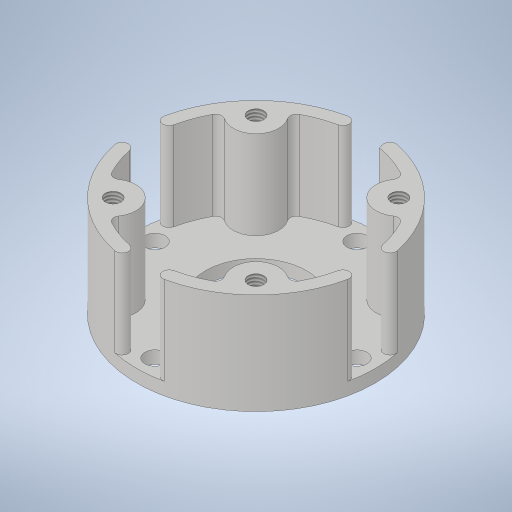
# Autodesk Inventor part: NEO MOUNT
Saved by Autodesk Inventor 2023.3 (Build 273359000, 359)
## iProperties
Created: 2024-01-28
Part Number: NEO MOUNT
Material: Generic
Document SubType Name: Modeling
Designer: mavericks
Density: 1 g/cm^3
Appearance: Default
Author: mavericks
Autodesk Inventor part; units mm, degrees
ref_plane "YZ Plane" through (0, 0, 0) normal (1, 0, 0) x (0, 1, 0)
ref_plane "XZ Plane" through (0, 0, 0) normal (0, 1, 0) x (-1, 0, 0)
ref_plane "XY Plane" through (0, 0, 0) normal (0, 0, 1) x (1, 0, 0)
sketch "Sketch1" plane through (0, 0, 0) normal (0, 1, 0) x (-1, 0, 0)
  circle A0 centre (0, 0) radius 25.4
  circle A1 centre (0, 0) radius 29.972
  dimension "d0" = 50.8
  dimension "d1" = 59.944
  constraints: 2 centre point, 2 coincident
  measures "d0" diameter of A0
  measures "d1" diameter of A1
extrude "Extrusion1" add sketch "Sketch1" along normal blind 3.175 contours A0 | A1
sketch "Sketch2" plane through (0, 3.175, 0) normal (0, 1, 0) x (1, 0, 0)
  circle A0 centre (0, 0) radius 25.4
  point P0 (-25.4, 0)
  point P1 (-17.9605, -17.9605)
  point P2 (0, -25.4)
  point P3 (17.9605, -17.9605)
  point P4 (25.4, 0)
  point P5 (17.9605, 17.9605)
  point P6 (0, 25.4)
  point P7 (-17.9605, 17.9605)
  dimension "d4" = 50.8
  dimension "d7" = 360
  constraints: 2 horizontal alignment, 1 coincident, 11 other
hole "Hole1" at (-25.4, 3.175, 0) at (0, 3.175, 25.4) at (25.4, 3.175, 0) at (0, 3.175, -25.4) direction (0, -1, 0) diameter 5.1054 end through all clearance for "Flat Head Machine Screw (82)" size "#10" standard "Ansi Unified Screw Threads"
sketch "Sketch3" plane through (0, 3.175, 0) normal (0, 1, 0) x (1, 0, 0)
  circle A0 centre (0, 0) radius 29.972 projected
  circle A1 centre (0, 0) radius 26.797
  circle A2 centre (-17.9605, -17.9605) radius 5.7277
  circle A3 centre (-17.9605, 17.9605) radius 5.7277
  circle A4 centre (17.9605, 17.9605) radius 5.7277
  circle A5 centre (17.9605, -17.9605) radius 5.7277
  circle A6 centre (25.4, 0) radius 2.5527 projected
  circle A7 centre (-25.4, 0) radius 2.5527 projected
  circle A8 centre (0, -25.4) radius 2.5527 projected
  circle A9 centre (0, 25.4) radius 2.5527 projected
  circle A10 centre (0, 0) radius 29.972 projected
  point P0 (-22.5303, -14.5074)
  point P1 (-22.5303, 14.5074)
  point P2 (-14.5074, 22.5303)
  point P3 (14.5074, 22.5303)
  point P4 (22.5303, 14.5074)
  point P5 (22.5303, -14.5074)
  point P6 (14.5074, -22.5303)
  point P7 (-14.5074, -22.5303)
  point P8 (-26.7071, -2.1926)
  point P9 (-26.7071, 2.1926)
  point P10 (-2.1926, 26.7071)
  point P11 (2.1926, 26.7071)
  point P12 (26.7071, 2.1926)
  point P13 (26.7071, -2.1926)
  point P14 (2.1926, -26.7071)
  point P15 (-2.1926, -26.7071)
  dimension "d16" = 3.175
  constraints: 5 centre point
  measures "d16" radial gap between concentric circles of A0 A1
extrude "Extrusion2" add sketch "Sketch3" along normal blind 22.225 contours A0 A5 A1 A6 A4 | A4 A1 A0 | A0 A5 A1 | A4 A1 A9 A3 A0 | A0 A2 A1 A8 A5 | A3 A1 A0 | A1 A4 | A0 A2 A1 | A5 A1 | A3 A1 A7 A2 A0 | A3 A1 | A1 A2
sketch "Sketch4" plane through (0, 25.4, 0) normal (0, 1, 0) x (1, 0, 0)
  circle A0 centre (0, 0) radius 29.972 construction
  arc A1 (-26.7071, -2.1926) -> (-22.5303, -14.5074) centre (0, 0) ccw construction
  arc A2 (-26.7071, 2.1926) -> (-26.7071, -2.1926) centre (-25.4, 0) ccw construction
  arc A3 (-22.5303, 14.5074) -> (-26.7071, 2.1926) centre (0, 0) ccw construction
  arc A4 (-22.5303, 14.5074) -> (-14.5074, 22.5303) centre (-17.9605, 17.9605) ccw construction
  arc A5 (-2.1926, 26.7071) -> (-14.5074, 22.5303) centre (0, 0) ccw construction
  arc A6 (2.1926, 26.7071) -> (-2.1926, 26.7071) centre (0, 25.4) ccw construction
  arc A7 (14.5074, 22.5303) -> (2.1926, 26.7071) centre (0, 0) ccw construction
  arc A8 (14.5074, 22.5303) -> (22.5303, 14.5074) centre (17.9605, 17.9605) ccw construction
  arc A9 (26.7071, 2.1926) -> (22.5303, 14.5074) centre (0, 0) ccw construction
  arc A10 (26.7071, -2.1926) -> (26.7071, 2.1926) centre (25.4, 0) ccw construction
  arc A11 (22.5303, -14.5074) -> (26.7071, -2.1926) centre (0, 0) ccw construction
  arc A12 (22.5303, -14.5074) -> (14.5074, -22.5303) centre (17.9605, -17.9605) ccw construction
  arc A13 (2.1926, -26.7071) -> (14.5074, -22.5303) centre (0, 0) ccw construction
  arc A14 (-2.1926, -26.7071) -> (2.1926, -26.7071) centre (0, -25.4) ccw construction
  arc A15 (-14.5074, -22.5303) -> (-2.1926, -26.7071) centre (0, 0) ccw construction
  arc A16 (-14.5074, -22.5303) -> (-22.5303, -14.5074) centre (-17.9605, -17.9605) ccw construction
  arc A17 (26.7071, 2.1926) -> (22.5303, 14.5074) centre (0, 0) ccw construction
  arc A18 (14.5074, 22.5303) -> (22.5303, 14.5074) centre (17.9605, 17.9605) ccw construction
  arc A19 (14.5074, 22.5303) -> (2.1926, 26.7071) centre (0, 0) ccw construction
  arc A20 (-2.1926, 26.7071) -> (2.1926, 26.7071) centre (0, 25.4) ccw construction
  arc A21 (-2.1926, 26.7071) -> (-14.5074, 22.5303) centre (0, 0) ccw construction
  arc A22 (-22.5303, 14.5074) -> (-14.5074, 22.5303) centre (-17.9605, 17.9605) ccw construction
  arc A23 (-22.5303, 14.5074) -> (-26.7071, 2.1926) centre (0, 0) ccw construction
  arc A24 (-26.7071, -2.1926) -> (-26.7071, 2.1926) centre (-25.4, 0) ccw construction
  arc A25 (-26.7071, -2.1926) -> (-22.5303, -14.5074) centre (0, 0) ccw construction
  arc A26 (-14.5074, -22.5303) -> (-22.5303, -14.5074) centre (-17.9605, -17.9605) ccw construction
  arc A27 (-14.5074, -22.5303) -> (-2.1926, -26.7071) centre (0, 0) ccw construction
  arc A28 (2.1926, -26.7071) -> (-2.1926, -26.7071) centre (0, -25.4) ccw construction
  arc A29 (2.1926, -26.7071) -> (14.5074, -22.5303) centre (0, 0) ccw construction
  arc A30 (22.5303, -14.5074) -> (14.5074, -22.5303) centre (17.9605, -17.9605) ccw construction
  arc A31 (22.5303, -14.5074) -> (26.7071, -2.1926) centre (0, 0) ccw construction
  arc A32 (26.7071, 2.1926) -> (26.7071, -2.1926) centre (25.4, 0) ccw construction
  circle A33 centre (-25.4, 0) radius 4.7625
  circle A34 centre (0, 25.4) radius 4.7625
  circle A35 centre (25.4, 0) radius 4.7625
  circle A36 centre (0, -25.4) radius 4.7625
  dimension "d34" = 9.525
  dimension "d35" = 9.525
  dimension "d36" = 9.525
  dimension "d37" = 9.525
  constraints: 4 centre point, 4 coincident
  measures "d34" diameter of A33
  measures "d35" diameter of A34
  measures "d36" diameter of A35
  measures "d37" diameter of A36
hole "Hole2" at (-17.9605, 25.4, -17.9605) at (-17.9605, 25.4, 17.9605) at (17.9605, 25.4, 17.9605) at (17.9605, 25.4, -17.9605) direction (0, -1, 0) diameter 3.9624 end through all thread size "10-32 UNF" class "2B" standard "ANSI Unified Screw Threads"
extrude "Extrusion3" cut sketch "Sketch4" against normal up to surface (22.225 mm away)
fillet "Fillet1" radius 1.5875 23 edges at (-29.937, 14.2875, -1.4481) (-26.3889, 14.2875, -4.6587) (-1.4481, 14.2875, -29.937) (1.4481, 14.2875, -29.937) (-4.6587, 14.2875, -26.3889) (-14.5074, 14.2875, -22.5303) (-22.5303, 14.2875, -14.5074) (22.5303, 14.2875, -14.5074) (14.5074, 14.2875, -22.5303) (29.937, 14.2875, -1.4481) (26.3889, 14.2875, -4.6587) (29.937, 14.2875, 1.4481) (26.3889, 14.2875, 4.6587) (22.5303, 14.2875, 14.5074) (14.5074, 14.2875, 22.5303) (4.6587, 14.2875, 26.3889) (-4.6587, 14.2875, 26.3889) (-1.4481, 14.2875, 29.937) (1.4481, 14.2875, 29.937) (-14.5074, 14.2875, 22.5303) (-22.5303, 14.2875, 14.5074) (-26.3889, 14.2875, 4.6587) (-29.937, 14.2875, 1.4481)
sketch "Sketch5" plane through (0, 3.175, 0) normal (0, 1, 0) x (1, 0, 0)
  circle A0 centre (0, 0) radius 25.5016 construction
  circle A1 centre (0, 0) radius 12.7
  dimension "d41" = 51.0032
  dimension "d42" = 25.4
  constraints: 2 centre point, 2 coincident
  measures "d41" diameter of A0
  measures "d42" diameter of A1
extrude "Extrusion4" cut sketch "Sketch5" against normal through all
equation "\"d35\" = d34"
equation "\"d36\" = d34"
equation "\"d37\" = d34"
body "Solid1"
